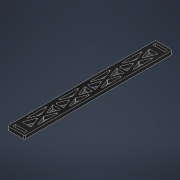
# Autodesk Inventor part: mount_battery_fastener
Saved by Autodesk Inventor 2021 (Build 250183000, 183)
## iProperties
Created: 2021-01-30
Part Number: mount_battery_fastener
Material: ABS Plastic
Document SubType Name: Modeling
Designer: User
Density: 1.06 g/cm^3
Appearance: Smooth - Black
Author: User
Autodesk Inventor part; units mm, degrees
ref_plane "YZ Plane" through (0, 0, 0) normal (1, 0, 0) x (0, 1, 0)
ref_plane "XZ Plane" through (0, 0, 0) normal (0, 1, 0) x (-1, 0, 0)
ref_plane "XY Plane" through (0, 0, 0) normal (0, 0, 1) x (1, 0, 0)
sketch "Sketch1" plane through (0, 0, 0) normal (0, 1, 0) x (-1, 0, 0)
  line L0 (-6.8, 0) -> (-6.8, 55.5)
  line L1 (-5.8, 56.5) -> (5.8, 56.5)
  line L2 (6.8, 55.5) -> (6.8, 0)
  line L3 (0, 0) -> (0, 56.5) construction
  line L4 (-4.8, 52.5) -> (4.8, 52.5)
  line L5 (4.8, 52.5) -> (4.8, 54.5)
  line L6 (4.8, 54.5) -> (-4.8, 54.5)
  line L7 (-4.8, 54.5) -> (-4.8, 52.5)
  arc A0 (-5.8, 56.5) -> (-6.8, 55.5) centre (-5.8, 55.5) ccw
  arc A1 (6.8, 55.5) -> (5.8, 56.5) centre (5.8, 55.5) ccw
  line L8 (6.8, 0) -> (-6.8, 0) construction
  line L9 (4.8, 48.5) -> (-4.8, 48.5)
  line L10 (4.8, 48.5) -> (4.8, 0)
  line L11 (-4.8, 48.5) -> (-4.8, 0)
  line L12 (4.8, 48.5) -> (-4.8, 24.25) construction
  line L13 (4.8, 0) -> (-4.8, 24.25) construction
  line L14 (-4.8, 0) -> (4.8, 24.25) construction
  line L15 (-4.8, 48.5) -> (4.8, 24.25) construction
  line L16 (-4.8, 24.25) -> (4.8, 24.25) construction
  line L17 (4.8, 2.7168) -> (1.0755, 12.125)
  line L18 (1.0755, 12.125) -> (4.8, 21.5332)
  line L19 (4.8, 26.9668) -> (1.0755, 36.375)
  line L20 (1.0755, 36.375) -> (4.8, 45.7832)
  line L21 (-1.0755, 36.375) -> (-4.8, 26.9668)
  line L22 (-1.0755, 36.375) -> (-4.8, 45.7832)
  line L23 (3.3286, 23.25) -> (0, 14.8418)
  line L24 (0, 14.8418) -> (-3.3286, 23.25)
  line L25 (-3.3286, 23.25) -> (3.3286, 23.25)
  line L26 (3.3286, 25.25) -> (-3.3286, 25.25)
  line L27 (-3.3286, 25.25) -> (0, 33.6582)
  line L28 (0, 33.6582) -> (3.3286, 25.25)
  line L29 (-1.0755, 12.125) -> (-4.8, 2.7168)
  line L30 (-1.0755, 12.125) -> (-4.8, 21.5332)
  line L31 (0, 39.0918) -> (3.7245, 48.5)
  line L32 (0, 39.0918) -> (-3.7245, 48.5)
  line L33 (3.3286, 1) -> (-3.3286, 1)
  line L34 (-3.3286, 1) -> (0, 9.4082)
  line L35 (3.3286, 1) -> (0, 9.4082)
  line L36 (-6.8, 0) -> (-6.8, -55.5)
  line L37 (-5.8, -56.5) -> (5.8, -56.5)
  line L38 (6.8, -55.5) -> (6.8, 0)
  line L39 (-4.8, -52.5) -> (4.8, -52.5)
  line L40 (4.8, -52.5) -> (4.8, -54.5)
  line L41 (4.8, -54.5) -> (-4.8, -54.5)
  line L42 (-4.8, -54.5) -> (-4.8, -52.5)
  arc A2 (-6.8, -55.5) -> (-5.8, -56.5) centre (-5.8, -55.5) ccw
  arc A3 (5.8, -56.5) -> (6.8, -55.5) centre (5.8, -55.5) ccw
  line L43 (4.8, -48.5) -> (-4.8, -48.5)
  line L44 (4.8, -48.5) -> (4.8, 0)
  line L45 (-4.8, -48.5) -> (-4.8, 0)
  line L46 (4.8, -48.5) -> (-4.8, -24.25) construction
  line L47 (4.8, 0) -> (-4.8, -24.25) construction
  line L48 (-4.8, 0) -> (4.8, -24.25) construction
  line L49 (-4.8, -48.5) -> (4.8, -24.25) construction
  line L50 (-4.8, -24.25) -> (4.8, -24.25) construction
  line L51 (4.8, -2.7168) -> (1.0755, -12.125)
  line L52 (1.0755, -12.125) -> (4.8, -21.5332)
  line L53 (4.8, -26.9668) -> (1.0755, -36.375)
  line L54 (1.0755, -36.375) -> (4.8, -45.7832)
  line L55 (-1.0755, -36.375) -> (-4.8, -26.9668)
  line L56 (-1.0755, -36.375) -> (-4.8, -45.7832)
  line L57 (3.3286, -23.25) -> (0, -14.8418)
  line L58 (0, -14.8418) -> (-3.3286, -23.25)
  line L59 (-3.3286, -23.25) -> (3.3286, -23.25)
  line L60 (3.3286, -25.25) -> (-3.3286, -25.25)
  line L61 (-3.3286, -25.25) -> (0, -33.6582)
  line L62 (0, -33.6582) -> (3.3286, -25.25)
  line L63 (-1.0755, -12.125) -> (-4.8, -2.7168)
  line L64 (-1.0755, -12.125) -> (-4.8, -21.5332)
  line L65 (0, -39.0918) -> (3.7245, -48.5)
  line L66 (0, -39.0918) -> (-3.7245, -48.5)
  line L67 (3.3286, -1) -> (-3.3286, -1)
  line L68 (-3.3286, -1) -> (0, -9.4082)
  line L69 (3.3286, -1) -> (0, -9.4082)
  point P0 (-6.8, 56.5)
  point P1 (6.8, 56.5)
  point P2 (0, 0)
  point P3 (-6.8, -56.5)
  point P4 (6.8, -56.5)
  point P5 (0, -56.5)
  dimension "d6" = 13.6
  dimension "d10" = 2
  dimension "d11" = 1
  dimension "d12" = 2
  dimension "d15" = 9.6
  dimension "d16" = 52.5
  dimension "d17" = 4
  dimension "d21" = 2
  dimension "d22" = 2
  dimension "d23" = 2
  dimension "d25" = 2
  dimension "d26" = 2
  dimension "d28" = 2
  dimension "d29" = 2
  dimension "d30" = 2
  dimension "d31" = 2
  dimension "d32" = 2
  dimension "d33" = 2
  dimension "d38" = 2
  dimension "d39" = 2
  dimension "d40" = 2
  dimension "d41" = 2
  dimension "d42" = 2
  dimension "d43" = 2
  constraints: 140 end point, 41 symmetric about line, 31 point on line, 20 parallel, 8 point on circle, 7 midpoint, 5 horizontal, 5 perpendicular, 4 centre point, 4 horizontal alignment, 4 tangent, 2 vertical alignment, 1 equal length, 1 equal radius, 1 vertical, 4 other
  measures "d6" distance of point (-6.8, 56.5) point (6.8, 56.5)
  measures "d10" distance between parallel lines of L1 L6
  measures "d11" radius of A0
  measures "d12" distance between parallel lines of L4 L6
  measures "d15" distance of L4.start L4.end
  measures "d16" distance from line of L3.start L4
  measures "d17" distance between parallel lines of L9 L4
  measures "d21" distance between parallel lines of L0 L11
  measures "d22" distance between parallel lines of L2 L10
  measures "d23" diameter of L17 L13
  measures "d25" diameter of L18 L14
  measures "d26" diameter of L23 L14
  measures "d28" diameter of L29 L14
  measures "d29" diameter of L25 L16
  measures "d30" diameter of L26 L16
  measures "d31" diameter of L28 L15
  measures "d32" diameter of L19 L15
  measures "d33" diameter of L20 L12
  measures "d38" diameter of L22 L15
  measures "d39" diameter of L21 L12
  measures "d40" diameter of L32 L15
  measures "d41" diameter of L30 L13
  measures "d42" diameter of L33 L8
  measures "d43" diameter of L35 L13
extrude "Extrusion2" add sketch "Sketch1" along normal blind 2.6 contours L0 A0 L1 A1 L2 L38 A3 L37 A2 L36 | L10 L20 L19 L18 L17 L44 L51 L52 L53 L54 L43 L65 L66 L45 L56 L55 L64 L63 L11 L29 L30 L21 L22 L9 L32 L31
fillet "Fillet1" radius 0.4 47 edges at (-4.8, 1.3, 45.7832) (-4.8, 1.3, 26.9668) (-1.0755, 1.3, 36.375) (-3.7245, 1.3, 48.5) (0, 1.3, 39.0918) (3.7245, 1.3, 48.5) (4.8, 1.3, 45.7832) (1.0755, 1.3, 36.375) (0, 1.3, 33.6582) (3.3286, 1.3, 25.25) (4.8, 1.3, 26.9668) (3.3286, 1.3, 23.25) (-3.3286, 1.3, 23.25) (-4.8, 1.3, 21.5332) (0, 1.3, 14.8418) (-1.0755, 1.3, 12.125) (3.3286, 1.3, 1) (-3.3286, 1.3, 1) (-4.8, 1.3, 2.7168) (0, 1.3, 9.4082) (1.0755, 1.3, 12.125) (4.8, 1.3, 2.7168) (4.8, 1.3, 21.5332) (-3.3286, 1.3, -1) (0, 1.3, -9.4082) (3.3286, 1.3, -1) (4.8, 1.3, -2.7168) (1.0755, 1.3, -12.125) (-1.0755, 1.3, -12.125) (-4.8, 1.3, -2.7168) (-4.8, 1.3, -21.5332) (-3.3286, 1.3, -23.25) (3.3286, 1.3, -23.25) (0, 1.3, -14.8418) (4.8, 1.3, -21.5332) (-3.3286, 1.3, -25.25) (0, 1.3, -33.6582) (3.3286, 1.3, -25.25) (4.8, 1.3, -26.9668) (1.0755, 1.3, -36.375) (4.8, 1.3, -45.7832) (3.7245, 1.3, -48.5) (-3.7245, 1.3, -48.5) (0, 1.3, -39.0918) (-4.8, 1.3, -45.7832) (-4.8, 1.3, -26.9668) (-1.0755, 1.3, -36.375)
equation "\"d21\" = link_width"
equation "\"d22\" = link_width"
equation "\"d23\" = link_width"
equation "\"d25\" = link_width"
equation "\"d26\" = link_width"
equation "\"d28\" = link_width"
equation "\"d29\" = link_width"
equation "\"d30\" = link_width"
equation "\"d31\" = link_width"
equation "\"d32\" = link_width"
equation "\"d33\" = link_width"
equation "\"d38\" = link_width"
equation "\"d39\" = link_width"
equation "\"d40\" = link_width"
equation "\"d41\" = link_width"
equation "\"d42\" = link_width"
equation "\"d43\" = link_width"
equation "\"link_width\" = 2"
body "Solid2"
